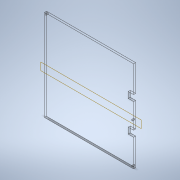
# Autodesk Inventor part: CoverPSU
Saved by Autodesk Inventor 2022.2 (Build 262287000, 287)
## iProperties
Created: 2022-01-15
Part Number: CoverPSU
Material: Generic
Document SubType Name: Modeling
Designer: siwat
Density: 1 g/cm^3
Appearance: Default
Author: siwat
Autodesk Inventor part; units mm, degrees
ref_plane "YZ Plane" through (0, 0, 0) normal (1, 0, 0) x (0, 1, 0)
ref_plane "XZ Plane" through (0, 0, 0) normal (0, 1, 0) x (-1, 0, 0)
ref_plane "XY Plane" through (0, 0, 0) normal (0, 0, 1) x (1, 0, 0)
ref_plane "Work Plane1" through (0, 0, 0) normal (0, 0, 1) x (1, 0, 0)
sketch "Sketch1" plane through (0, 0, 0) normal (0, 0, 1) x (1, 0, 0)
  line L0 (66.5748, -56.8802) -> (-66.4252, -56.8802)
  line L1 (-66.4252, -56.8802) -> (-66.4252, 79.1198)
  line L2 (-66.4252, 79.1198) -> (66.5748, 79.1198)
  line L3 (66.5748, 79.1198) -> (66.5748, -56.8802)
  circle A0 centre (64.4766, 5.0982) radius 1
  circle A1 centre (-64.6107, 77.1629) radius 1
  circle A2 centre (64.6335, -54.3469) radius 1
  point P0 (0, 0)
  dimension "d0" = 2
  dimension "d1" = 2
  dimension "d4" = 2
  dimension "d11" = 136
  dimension "d12" = 133
  constraints: 8 end point, 3 centre point, 2 parallel, 1 horizontal, 1 perpendicular
  measures "d0" diameter of A0
  measures "d1" diameter of A1
  measures "d4" diameter of A2
  measures "d11" distance of L2.end L0.start
  measures "d12" distance of L1.end L2.end
extrude "Extrusion1" add sketch "Sketch1" along normal blind 3
sketch "Sketch2" plane through (0, 0, 3) normal (0, 0, 1) x (1, 0, 0)
  line L0 (66.5748, -56.8802) -> (66.5748, 79.1198) projected
  line L1 (66.5748, -15.8467) -> (58.5748, -15.8467)
  line L2 (58.5748, -15.8467) -> (58.5748, -6.8467)
  line L3 (58.5748, -6.8467) -> (66.5748, -6.8467)
  line L4 (66.5748, -6.8467) -> (66.5748, -15.8467)
  line L5 (66.5748, 30.2369) -> (58.5748, 30.2369)
  line L6 (58.5748, 30.2369) -> (58.5748, 39.2369)
  line L7 (58.5748, 39.2369) -> (66.5748, 39.2369)
  line L8 (66.5748, 39.2369) -> (66.5748, 30.2369)
  point P0 (0, 0)
  point P1 (66.5748, 39.2369)
  dimension "d5" = 8
  dimension "d6" = 9
  dimension "d7" = 8
  dimension "d8" = 9
  constraints: 16 end point, 4 parallel, 2 horizontal, 2 perpendicular, 2 point on line
  measures "d5" distance of L2.end L3.end
  measures "d6" distance of L1.end L2.end
  measures "d7" distance of L6.end L7.end
  measures "d8" distance of L5.end L6.end
extrude "Extrusion2" cut sketch "Sketch2" against normal through all
body "Solid1"
